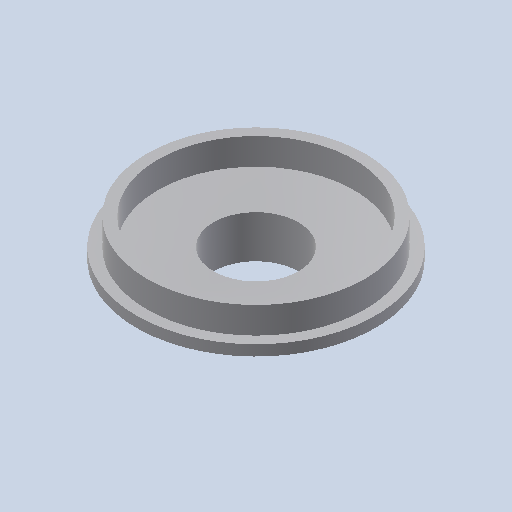
# Autodesk Inventor part: Pieza 1.2 final
Saved by Autodesk Inventor 2023.1 (Build 271208000, 208)
## iProperties
Created: 2022-10-20
Part Number: Pieza 1.2 final
Material: ABS Plastic
Document SubType Name: Modeling
Designer: User
Density: 1.06 g/cm^3
Appearance: Smooth - White
Author: User
Autodesk Inventor part; units mm, degrees
ref_plane "YZ Plane" through (0, 0, 0) normal (1, 0, 0) x (0, 1, 0)
ref_plane "XZ Plane" through (0, 0, 0) normal (0, 1, 0) x (-1, 0, 0)
ref_plane "XY Plane" through (0, 0, 0) normal (0, 0, 1) x (1, 0, 0)
sketch "Sketch1" plane through (0, 0, 0) normal (0, 1, 0) x (-1, 0, 0)
  circle A0 centre (0, 0) radius 22.5
  dimension "d0" = 45
  constraints: 1 centre point, 1 coincident
  measures "d0" diameter of A0
extrude "Extrusion1" add sketch "Sketch1" along normal blind 2
sketch "Sketch2" plane through (0, 2, 0) normal (0, 1, 0) x (1, 0, 0)
  circle A0 centre (0, 0) radius 22.5 projected
  circle A1 centre (0, 0) radius 20.5
  circle A2 centre (0, 0) radius 18.5
  dimension "d3" = 2
  dimension "d4" = 4
  constraints: 2 centre point
  measures "d3" radial gap between concentric circles of A0 A1
  measures "d4" radial gap between concentric circles of A0 A2
extrude "Extrusion2" add sketch "Sketch2" along normal blind 5 contours A1
sketch "Sketch3" plane through (0, 0, 0) normal (0, -1, 0) x (1, 0, 0)
  circle A0 centre (0, 0) radius 20.5 projected
  circle A1 centre (0, 0) radius 22.5 projected
  circle A2 centre (0, 0) radius 8
  dimension "d7" = 16
  constraints: 1 centre point, 1 coincident
  measures "d7" diameter of A2
extrude "Extrusion3" cut sketch "Sketch3" against normal blind 3 contours A2
sketch "Sketch4" plane through (0, 0, 0) normal (0, -1, 0) x (1, 0, 0)
  circle A0 centre (0, 0) radius 8 projected
  circle A1 centre (0, 0) radius 22.5 projected
  circle A2 centre (0, 0) radius 8 projected
  circle A3 centre (0, 0) radius 10
  dimension "d10" = 2
  constraints: 1 centre point
  measures "d10" radial gap between concentric circles of A0 A3
extrude "Extrusion4" add sketch "Sketch4" along normal blind 6 contours A3
body "Solid1"
